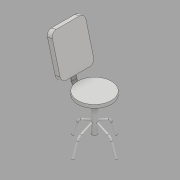
# Autodesk Inventor part: Chair_Orientation_Rest
Saved by Autodesk Inventor 2019.1 (Build 231200000, 200)
## iProperties
Created: 2018-10-29
Part Number: Chair_Orientation_Rest
Material: Generic
Document SubType Name: Modeling
Designer: t_gc
Density: 1 g/cm^3
Appearance: Default
Author: t_gc
Autodesk Inventor part; units mm, degrees
ref_plane "YZ Plane" through (0, 0, 0) normal (1, 0, 0) x (0, 1, 0)
sketch "Sketch1" plane through (0, 0, 0) normal (0, 0, 1) x (1, 0, 0)
  circle A0 centre (0, 0) radius 7.5
  dimension "d0" = 15
  constraints: 1 centre point, 1 coincident
  measures "d0" diameter of A0
extrude "Extrusion1" add sketch "Sketch1" along normal blind 100
sketch "Sketch2" plane through (0, 0, 100) normal (0, 0, 1) x (1, 0, 0)
  circle A0 centre (0, 0) radius 50
  dimension "d3" = 100
  constraints: 1 centre point, 1 coincident
  measures "d3" diameter of A0
extrude "Extrusion2" add sketch "Sketch2" along normal blind 10
sketch "Sketch3" plane through (0, 0, 0) normal (1, 0, 0) x (0, 1, 0)
  line L0 (-7.5, 0) -> (7.5, 0) projected
  line L1 (7.5, 0) -> (7.5, 100) projected
  arc A0 (50.3292, 5.6261) -> (40.3868, 16.5527) centre (32.5781, -0.5395) ccw
  line L2 (50.3292, 5.6261) -> (64.44, -35)
  line L3 (40.3868, 16.5527) -> (7.5, 31.5773)
  line L4 (7.5, 0) -> (7.5, 100) projected
  point P0 (0, 0)
  point P1 (0, 0)
  dimension "d14" = 64.44
  dimension "d15" = 35
  constraints: 4 end point, 2 point on circle, 2 tangent, 1 centre point, 1 coincident, 1 point on line
  measures "d14" horizontal distance of point (0, 0) L2.end
  measures "d15" vertical distance of point (0, 0) L2.end
ref_plane "Work Plane1" through (0, 64.44, -35) normal (0, 0.3281, -0.9446) x (-1, 0, 0)
sketch "Sketch4" plane through (0, 64.44, -35) normal (0, 0.3281, -0.9446) x (-1, 0, 0)
  circle A0 centre (0, 0) radius 2.5
  point P0 (0, -49.389)
  dimension "d7" = 5
  constraints: 1 centre point
  measures "d7" diameter of A0
sweep "Sweep1" add profiles "Sketch4" path "Sketch3" path curves L2 A0 L3
pattern_circular "Circular Pattern1" count 4 over 360 about axis through (0, 0, 0) along (0, 0, 1) of "Sweep1", "Extrusion1"
sketch "Sketch5" plane through (0, 0, 0) normal (1, 0, 0) x (0, 1, 0)
  line L0 (-50, 100) -> (50, 100) projected
  line L1 (-32.9907, 100) -> (-49.7498, 100)
  arc A0 (-60.5097, 108.3127) -> (-49.7498, 100) centre (-49.7498, 111.12) ccw
  line L2 (-60.5097, 108.3127) -> (-80.3043, 184.1803)
  point P0 (0, 0)
  constraints: 4 end point, 2 point on circle, 2 tangent, 1 centre point, 1 horizontal, 1 point on line
ref_plane "Work Plane2" through (0, -80.3043, 184.1803) normal (0, -0.2525, 0.9676) x (1, 0, 0)
sketch "Sketch6" plane through (0, -80.3043, 184.1803) normal (0, -0.2525, 0.9676) x (1, 0, 0)
  arc A0 (6.9669, -2.3182) -> (-6.7097, -2.3182) centre (0.1286, -20.1419) ccw
  arc A1 (7.95, 0.2444) -> (-7.6929, 0.2444) centre (0.1286, -20.1419) ccw
  arc A2 (-7.6929, 0.2444) -> (-6.7097, -2.3182) centre (-7.2013, -1.0369) ccw
  arc A3 (6.9669, -2.3182) -> (7.95, 0.2444) centre (7.4584, -1.0369) ccw
  point P0 (0, 31.2052)
  constraints: 8 point on circle, 4 centre point, 4 tangent
sweep "Sweep2" add profiles "Sketch6" path "Sketch5" path curves L2 A0 L1
ref_plane "Work Plane3" through (0.1286, -78.6659, 184.6078) normal (0, 0.9676, 0.2525) x (-1, 0, 0)
sketch "Sketch7" plane through (0.1286, -78.6659, 184.6078) normal (0, 0.9676, 0.2525) x (-1, 0, 0)
  line L0 (35, -60) -> (-35, -60)
  line L1 (-50, -45) -> (-50, 45)
  line L2 (-35, 60) -> (35, 60)
  line L3 (50, 45) -> (50, -45)
  line L4 (-7.8215, 0) -> (7.8215, 0) projected
  arc A0 (35, -60) -> (50, -45) centre (35, -45) ccw
  arc A1 (-50, -45) -> (-35, -60) centre (-35, -45) ccw
  arc A2 (50, 45) -> (35, 60) centre (35, 45) ccw
  arc A3 (-35, 60) -> (-50, 45) centre (-35, 45) ccw
  point P0 (0.1286, -198.4878)
  point P1 (-50, 60)
  point P2 (-50, -60)
  point P3 (50, 60)
  point P4 (0, 0)
  point P5 (0, 60)
  dimension "d18" = 60
  dimension "d19" = 120
  dimension "d20" = 100
  dimension "d21" = 15
  constraints: 8 end point, 8 point on circle, 8 tangent, 6 point on line, 4 centre point, 3 equal radius, 2 midpoint, 2 parallel, 1 horizontal, 1 perpendicular, 1 vertical alignment
  measures "d18" distance between parallel lines of L0 L4
  measures "d19" distance of point (-50, -60) point (-50, 60)
  measures "d20" distance of point (-50, 60) point (50, 60)
  measures "d21" radius of A0
extrude "Extrusion3" add sketch "Sketch7" along normal blind 15
body "Solid1"
